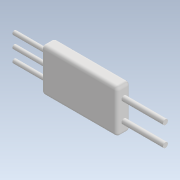
# Autodesk Inventor part: Esc_BlHeli_30A
Saved by Autodesk Inventor 2021.1 (Build 251245010, 245A)
## iProperties
Created: 2024-03-20
Part Number: Esc_BlHeli_30A
Material: Generic
Document SubType Name: Modeling
Designer: user
Mass: 29 g
Surface Area: 42.0726 cm^2
Volume: 9.95198 cm^3
Density: 2.91399 g/cm^3
Appearance: Galvanized
Author: user
Autodesk Inventor part; units mm, degrees
ref_plane "YZ Plane" through (0, 0, 0) normal (1, 0, 0) x (0, 1, 0)
ref_plane "XZ Plane" through (0, 0, 0) normal (0, 1, 0) x (-1, 0, 0)
ref_plane "XY Plane" through (0, 0, 0) normal (0, 0, 1) x (1, 0, 0)
sketch "Sketch1" plane through (0, 0, 0) normal (0, 0, 1) x (1, 0, 0)
  line L0 (0, 0) -> (-46, 0)
  line L1 (-46, 0) -> (-46, 26)
  line L2 (-46, 26) -> (0, 26)
  line L3 (0, 26) -> (0, 0)
  dimension "d0" = 46
  dimension "d1" = 26
  constraints: 8 end point, 2 parallel, 1 horizontal, 1 perpendicular
  measures "d0" distance of L1.end L2.end
  measures "d1" distance of L0.end L1.end
extrude "Extrusion1" add sketch "Sketch1" along normal blind 8
fillet "Fillet1" radius 2 12 edges at (-23, 26, 8) (-46, 13, 8) (-46, 26, 4) (0, 13, 8) (-23, 0, 8) (0, 26, 4) (0, 13, 0) (0, 0, 4) (-23, 0, 0) (-46, 0, 4) (-46, 13, 0) (-23, 26, 0)
sketch "Sketch2" plane through (0, 2, 6) normal (1, 0, 0) x (0, 0, -1)
  circle A0 centre (2, 17) radius 1.5
  line L0 (0, 0) -> (0, 22) projected
  line L1 (0, 22) -> (4, 22) projected
  line L2 (4, 22) -> (4, 0) projected
  line L3 (4, 0) -> (0, 0) projected
  circle A1 centre (2, 5) radius 1.5
  line L4 (2, 26.4217) -> (2, -4.8985)
  point P0 (6, -2)
  dimension "d5" = 3
  dimension "d6" = 3
  dimension "d7" = 5
  dimension "d8" = 5
  constraints: 2 centre point, 2 end point, 2 point on line, 1 parallel, 1 vertical
  measures "d5" diameter of A0
  measures "d6" diameter of A1
  measures "d7" distance from line of L3 A1.centre
  measures "d8" distance from line of L1 A0.centre
extrude "Extrusion2" add sketch "Sketch2" along normal blind 25 contours A0 L4 | L4 A0 | L4 A1 | A1 L4
sketch "Sketch3" plane through (-46, 2, 2) normal (-1, 0, 0) x (0, 0, 1)
  line L0 (4, 22) -> (4, 0) projected
  line L1 (0, 22) -> (4, 22) projected
  line L2 (0, 22) -> (4, 22) projected
  line L3 (0, 0) -> (0, 22) projected
  line L4 (4, 0) -> (0, 0) projected
  line L5 (4, 22) -> (4, 0) projected
  circle A0 centre (2, 18.2633) radius 1.25
  circle A1 centre (2, 10.9374) radius 1.25
  circle A2 centre (2, 3.4881) radius 1.25
  line L6 (2, 27.5735) -> (2, -5.6987)
  point P0 (-2, -2)
  dimension "d11" = 2.5
  dimension "d12" = 2.5
  dimension "d13" = 2.5
  constraints: 3 centre point, 2 end point, 2 midpoint, 2 point on line, 2 vertical
  measures "d11" diameter of A0
  measures "d12" diameter of A1
  measures "d13" diameter of A2
extrude "Extrusion3" add sketch "Sketch3" along normal blind 20 contours L6 A0 | A0 L6 | L6 A2 | A2 L6 | L6 A1 | A1 L6
body "Solid1"
